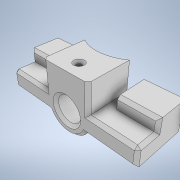
# Autodesk Inventor part: zad 8
Saved by Autodesk Inventor 2020 (Build 240168000, 168)
## iProperties
Created: 2022-04-10
Part Number: zad 8
Material: Ogólny
Document SubType Name: Modeling
Designer: likek
Density: 1 g/cm^3
Appearance: Domyślna
Author: likek
Autodesk Inventor part; units mm, degrees
ref_plane "YZ Plane" through (0, 0, 0) normal (1, 0, 0) x (0, 1, 0)
ref_plane "XZ Plane" through (0, 0, 0) normal (0, 1, 0) x (-1, 0, 0)
ref_plane "XY Plane" through (0, 0, 0) normal (0, 0, 1) x (1, 0, 0)
sketch "Szkic1" plane through (0, 0, 0) normal (0, 0, 1) x (1, 0, 0)
  arc A0 (-20.1556, -10) -> (20.1556, -10) centre (0, 0) ccw
  line L0 (-20.1556, -10) -> (-67, -10)
  line L1 (-67, -10) -> (-67, 8)
  line L2 (-67, 8) -> (-23, 8)
  line L3 (-23, 8) -> (-23, 36)
  line L4 (-23, 36) -> (23, 36)
  line L5 (23, 36) -> (23, 8)
  line L6 (23, 8) -> (67, 8)
  line L7 (67, 8) -> (67, -10)
  line L8 (67, -10) -> (20.1556, -10)
  point P0 (0, -22.5)
  dimension "d0" = 45
  dimension "d1" = 10
  dimension "d2" = 18
  dimension "d3" = 46
  dimension "d4" = 44
  dimension "d5" = 44
  dimension "d6" = 23
  dimension "d7" = 58.5
  constraints: 18 end point, 5 perpendicular, 3 point on circle, 3 point on line, 1 centre point, 1 coincident, 1 horizontal, 1 vertical
  measures "d0" diameter of A0
  measures "d1" distance from line of point (0, 0) L0
  measures "d2" distance of L0.end L1.end
  measures "d3" distance of L3.end L4.end
  measures "d4" distance of L1.end L2.end
  measures "d5" distance of L5.end L6.end
  measures "d6" horizontal distance of point (0, 0) L2.end
  measures "d7" distance from line of point (0, -22.5) L4
extrude "Wyciągnięcie proste1" add sketch "Szkic1" against normal blind 50
sketch "Szkic2" plane through (0, 0, 0) normal (0, 0, 1) x (1, 0, 0)
  circle A0 centre (0, 0) radius 12.5
  dimension "d10" = 25
  constraints: 1 centre point, 1 coincident
  measures "d10" diameter of A0
extrude "Wyciągnięcie proste2" cut sketch "Szkic2" against normal blind 50
sketch "Szkic3" plane through (23, 8, 0) normal (0, 1, 0) x (1, 0, 0)
  line L0 (0, 50) -> (44, 50) projected
  line L1 (44, 50) -> (9, 50)
  line L2 (9, 50) -> (9, 20)
  line L3 (9, 20) -> (44, 20)
  line L4 (44, 20) -> (44, 50)
  line L5 (-90, 50) -> (-46, 50) projected
  line L6 (-90, 50) -> (-55, 50)
  line L7 (-55, 50) -> (-55, 20)
  line L8 (-55, 20) -> (-90, 20)
  line L9 (-90, 20) -> (-90, 50)
  point P0 (-23, 0)
  point P1 (9, 50)
  dimension "d13" = 35
  dimension "d14" = 30
  dimension "d15" = 35
  dimension "d16" = 30
  constraints: 16 end point, 4 parallel, 2 horizontal, 2 perpendicular
  measures "d13" distance of L3.end L2.end
  measures "d14" distance of L2.end L1.end
  measures "d15" distance of L7.end L8.end
  measures "d16" distance of L6.end L7.end
extrude "Wyciągnięcie proste3" add sketch "Szkic3" along normal blind 12
sketch "Szkic4" plane through (-23, 36, 0) normal (0, 1, 0) x (1, 0, 0)
  circle A0 centre (23, 77.2029) radius 42
  point P0 (23, 0)
  point P1 (-9, 50)
  point P2 (55, 50)
  dimension "d19" = 84
  constraints: 2 point on circle, 1 centre point
  measures "d19" diameter of A0
extrude "Wyciągnięcie proste4" cut sketch "Szkic4" against normal blind 141.25
chamfer "Faza1" distance 3 angle 45 16 edges at (-45, 8, 0) (-23, 22, 0) (-67, 8, -10) (-67, 14, -20) (-49.5, 20, -20) (-67, -1, 0) (-43.5778, -10, 0) (0, -22.5, 0) (43.5778, -10, 0) (67, -1, 0) (45, 8, 0) (23, 22, 0) (67, 8, -10) (67, 14, -20) (49.5, 20, -20) (-12.5, 0, 0)
sketch "Szkic5" plane through (0, 36, -77.2029) normal (0, 1, 0) x (1, 0, 0)
  point P0 (0, -77.2029)
  point P1 (0, -63.2029)
  point P2 (161.096, 29.7407)
  dimension "d25" = 14
  measures "d25" distance of point (0, -63.203) point (0, -77.203)
hole "Otwór1" at (161.096, 36, -106.9437) at (0, 36, -14) direction (0, -1, 0) diameter 5.5 depth 23.81 tip angle 118 countersink diameter 10.4 countersink angle 90
